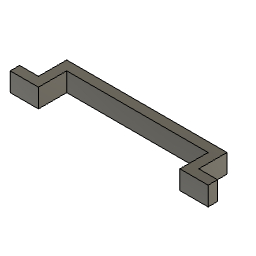
window holder v1 (Autodesk Fusion 360 design; units mm, degrees)
Autodesk Fusion 360 part; units mm, degrees
sketch "Sketch1" plane through (0, 0, 0) normal (0, 0, 1) x (1, 0, 0)
  line L0 (-50, 20) -> (35, 20)
  line L1 (35, 20) -> (35, 15)
  line L2 (35, 15) -> (-50, 15)
  line L3 (-50, 15) -> (-50, 20)
  line L4 (-50, 20) -> (-45, 20)
  line L5 (-45, 20) -> (-45, 0)
  line L6 (-45, 0) -> (-50, 0)
  line L7 (-50, 0) -> (-50, 20)
  line L8 (35, 20) -> (30, 20)
  line L9 (30, 20) -> (30, 0)
  line L10 (30, 0) -> (35, 0)
  line L11 (35, 0) -> (35, 20)
  line L12 (30, 0) -> (45, 0)
  line L13 (45, 0) -> (45, 5)
  line L14 (45, 5) -> (30, 5)
  line L15 (30, 5) -> (30, 0)
  line L16 (-45, 0) -> (-60, 0)
  line L17 (-60, 0) -> (-60, 5)
  line L18 (-60, 5) -> (-45, 5)
  line L19 (-45, 5) -> (-45, 0)
  dimension "d1" = 85
  dimension "d2" = 5
  dimension "d3" = 5
  dimension "d4" = 20
  dimension "d5" = 5
  dimension "d6" = 20
  dimension "d7" = 15
  dimension "d8" = 5
  dimension "d9" = 15
  dimension "d10" = 5
  constraint horizontal L0
  constraint vertical L1
  constraint horizontal L2
  constraint vertical L3
  constraint horizontal L4
  constraint vertical L5
  constraint horizontal L6
  constraint vertical L7
  constraint horizontal L8
  constraint vertical L9
  constraint horizontal L10
  constraint vertical L11
  constraint horizontal L12
  constraint vertical L13
  constraint horizontal L14
  constraint vertical L15
  constraint horizontal L16
  constraint vertical L17
  constraint horizontal L18
  constraint vertical L19
  measures "d1" distance of L0.start L0.end
  measures "d2" distance of L0.start L2.end
  measures "d3" distance of L0.start L4.end
  measures "d4" distance of L0.start L6.end
  measures "d5" distance of L0.end L8.end
  measures "d6" distance of L0.end L10.end
  measures "d7" distance of L9.end L12.end
  measures "d8" distance of L9.end L14.end
  measures "d9" distance of L5.end L16.end
  measures "d10" distance of L5.end L18.end
extrude "Extrude1" add sketch "Sketch1" along normal blind 10
